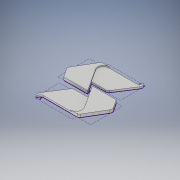
# Autodesk Inventor part: Segeco
Saved by Autodesk Inventor 2017 (Build 210142000, 142)
## iProperties
Created: 2019-09-05
Part Number: Segeco
Material: Generic
Document SubType Name: Modeling
Designer: Eduardo
Density: 1 g/cm^3
Appearance: Default
Author: Eduardo
Autodesk Inventor part; units mm, degrees
ref_plane "YZ Plane" through (0, 0, 0) normal (1, 0, 0) x (0, 1, 0)
ref_plane "XZ Plane" through (0, 0, 0) normal (0, 1, 0) x (-1, 0, 0)
ref_plane "XY Plane" through (0, 0, 0) normal (0, 0, 1) x (1, 0, 0)
sketch "SEGECO_Logo_A" plane through (0, 0, 0) normal (0, 0, 1) x (1, 0, 0)
  line L0 (106.4876, 54.7826) -> (93.1423, 75.2888)
  line L1 (131.2894, 54.7826) -> (106.4876, 54.7826)
  arc A0 (131.2894, 54.7826) -> (135.2032, 56.9315) centre (131.2894, 59.4212) ccw
  line L2 (101.453, 90.6131) -> (148.9397, 90.6131)
  arc A1 (101.453, 90.6131) -> (93.1423, 75.2888) centre (101.453, 80.6974) ccw
  line L3 (155.6383, 89.056) -> (135.2032, 56.9315)
  arc A2 (148.9397, 90.6131) -> (153.4753, 98.1434) centre (148.9397, 95.7441) ccw
  arc A3 (155.6383, 89.056) -> (153.4753, 98.1434) centre (150.146, 92.5498) ccw
  line L4 (91.5373, 98.1434) -> (156.6554, 98.1434) construction
  line L5 (156.6554, 98.1434) -> (156.6554, 54.7826) construction
  line L6 (156.6554, 54.7826) -> (91.5373, 54.7826) construction
  line L7 (91.5373, 54.7826) -> (91.5373, 98.1434) construction
  line L8 (148.9397, 90.6131) -> (148.9397, 98.1434) construction
  dimension "d53" = 9.9157
  dimension "d54" = 5.1311
  dimension "d55" = 6.5095
  dimension "d56" = 4.6386
  dimension "d63" = 1.2062
  dimension "d90" = 123.056
  dimension "d91" = 24.8018
  dimension "d92" = 20.5062
  dimension "d93" = 43.3608
  dimension "d95" = 65.1181
  measures "d53" radius of A1
  measures "d54" radius of A2
  measures "d55" radius of A3
  measures "d56" radius of A0
  measures "d63" distance from line of L8 A3.centre
  measures "d90" angle of L0 L1
  measures "d91" distance of L1.start L1.end
  measures "d92" distance from line of L0.end L6
  measures "d93" distance of L6.end L4.start
  measures "d95" distance of L4.start L4.end
sketch "SEGECO_Logo_B" plane through (0, 0, 0) normal (0, 0, 1) x (1, 0, 0)
  arc A0 (59.5618, 148.275) -> (51.2511, 132.9507) centre (59.5618, 138.3593) ccw
  line L0 (59.5618, 148.275) -> (48.761, 148.275)
  line L1 (45.0457, 146.1613) -> (26.0996, 114.2875)
  line L2 (26.2488, 108.0158) -> (35.65, 93.7862)
  line L3 (35.65, 93.7862) -> (76.7391, 93.7862)
  line L4 (76.7391, 93.7862) -> (51.2511, 132.9507)
  arc A1 (26.0996, 114.2875) -> (26.2488, 108.0158) centre (31.1752, 111.2706) ccw
  line L5 (25.2707, 148.275) -> (76.7391, 148.275) construction
  line L6 (76.7391, 148.275) -> (76.7391, 93.7862) construction
  line L7 (76.7391, 93.7862) -> (25.2707, 93.7862) construction
  line L8 (25.2707, 93.7862) -> (25.2707, 148.275) construction
  arc A2 (48.761, 148.275) -> (45.0457, 146.1613) centre (48.761, 143.9529) ccw
  point P0 (75.2707, 99.3568)
  dimension "d68" = 9.9157
  dimension "d70" = 5.9045
  dimension "d76" = 5.5706
  dimension "d77" = 1.4684
  dimension "d82" = 123.452
  dimension "d83" = 123.056
  dimension "d84" = 14.2295
  dimension "d86" = 54.4888
  dimension "d87" = 51.4684
  dimension "d89" = 23.4904
  dimension "d100" = 4.3221
  measures "d68" radius of A0
  measures "d70" radius of A1
  measures "d76" vertical distance of L3.end point (75.271, 99.357)
  measures "d77" distance from line of L6 point (75.271, 99.357)
  measures "d82" angle of L7 L2
  measures "d83" angle of L4 L7
  measures "d84" distance from line of L2.start L7
  measures "d86" distance of L7.end L5.start
  measures "d87" distance of L5.start L5.end
  measures "d89" distance of L5.start L0.end
  measures "d100" radius of A2
sketch "Logo_base" plane through (0, 0, 0) normal (0, 0, 1) x (1, 0, 0)
  arc A0 (-15.7088, 48.9181) -> (-24.0196, 33.5938) centre (-15.7088, 39.0024) ccw
  line L0 (-15.7088, 48.9181) -> (-26.5096, 48.9181)
  line L1 (-30.2249, 46.8044) -> (-49.171, 14.9307)
  line L2 (-49.0219, 8.6589) -> (-39.6206, -5.5706)
  line L3 (-39.6206, -5.5706) -> (1.4684, -5.5706)
  line L4 (1.4684, -5.5706) -> (-24.0196, 33.5938)
  arc A1 (-49.171, 14.9307) -> (-49.0219, 8.6589) centre (-44.0955, 11.9137) ccw
  line L5 (-50, 48.9181) -> (1.4684, 48.9181) construction
  line L6 (1.4684, 48.9181) -> (1.4684, -5.5706) construction
  line L7 (1.4684, -5.5706) -> (-50, -5.5706) construction
  line L8 (-50, -5.5706) -> (-50, 48.9181) construction
  arc A2 (-26.5096, 48.9181) -> (-30.2249, 46.8044) centre (-26.5096, 44.596) ccw
  line L9 (-10.6743, 13.0877) -> (-24.0196, 33.5938)
  line L10 (14.1275, 13.0877) -> (-10.6743, 13.0877)
  arc A3 (14.1275, 13.0877) -> (18.0413, 15.2366) centre (14.1275, 17.7263) ccw
  line L11 (-15.7088, 48.9181) -> (31.7778, 48.9181)
  arc A4 (-15.7088, 48.9181) -> (-24.0196, 33.5938) centre (-15.7088, 39.0024) ccw
  line L12 (38.4765, 47.361) -> (18.0413, 15.2366)
  arc A5 (31.7778, 48.9181) -> (36.3134, 56.4485) centre (31.7778, 54.0492) ccw
  arc A6 (38.4765, 47.361) -> (36.3134, 56.4485) centre (32.9841, 50.8548) ccw
  line L13 (-25.6245, 56.4485) -> (39.4935, 56.4485) construction
  line L14 (39.4935, 56.4485) -> (39.4935, 13.0877) construction
  line L15 (39.4935, 13.0877) -> (-25.6245, 13.0877) construction
  line L16 (-25.6245, 13.0877) -> (-25.6245, 56.4485) construction
  line L17 (31.7778, 48.9181) -> (31.7778, 56.4485) construction
  arc A7 (15.7088, -48.9181) -> (24.0196, -33.5938) centre (15.7088, -39.0024) ccw
  line L18 (15.7088, -48.9181) -> (26.5096, -48.9181)
  line L19 (30.2249, -46.8044) -> (49.171, -14.9307)
  line L20 (49.0219, -8.6589) -> (39.6206, 5.5706)
  line L21 (39.6206, 5.5706) -> (-1.4684, 5.5706)
  line L22 (-1.4684, 5.5706) -> (24.0196, -33.5938)
  arc A8 (49.171, -14.9307) -> (49.0219, -8.6589) centre (44.0955, -11.9137) ccw
  line L23 (50, -48.9181) -> (-1.4684, -48.9181) construction
  line L24 (-1.4684, -48.9181) -> (-1.4684, 5.5706) construction
  line L25 (-1.4684, 5.5706) -> (50, 5.5706) construction
  line L26 (50, 5.5706) -> (50, -48.9181) construction
  arc A9 (26.5096, -48.9181) -> (30.2249, -46.8044) centre (26.5096, -44.596) ccw
  line L27 (10.6743, -13.0877) -> (24.0196, -33.5938)
  line L28 (-14.1275, -13.0877) -> (10.6743, -13.0877)
  arc A10 (-14.1275, -13.0877) -> (-18.0413, -15.2366) centre (-14.1275, -17.7263) ccw
  line L29 (15.7088, -48.9181) -> (-31.7778, -48.9181)
  arc A11 (15.7088, -48.9181) -> (24.0196, -33.5938) centre (15.7088, -39.0024) ccw
  line L30 (-38.4765, -47.361) -> (-18.0413, -15.2366)
  arc A12 (-31.7778, -48.9181) -> (-36.3134, -56.4485) centre (-31.7778, -54.0492) ccw
  arc A13 (-38.4765, -47.361) -> (-36.3134, -56.4485) centre (-32.9841, -50.8548) ccw
  line L31 (25.6245, -56.4485) -> (-39.4935, -56.4485) construction
  line L32 (-39.4935, -56.4485) -> (-39.4935, -13.0877) construction
  line L33 (-39.4935, -13.0877) -> (25.6245, -13.0877) construction
  line L34 (25.6245, -13.0877) -> (25.6245, -56.4485) construction
  line L35 (-31.7778, -48.9181) -> (-31.7778, -56.4485) construction
  point P0 (0, 0)
  constraints: 2 other
extrude "Logo_A" add sketch "Logo_base" along normal blind 3 contours L11 A5 A6 L12 A3 L10 L4 A0 | L29 A12 A13 L30 A10 L28 L22 A7
extrude "Logo_B" add sketch "Logo_base" along normal blind 5 contours A0 L4 L3 L2 A1 L1 A2 L0 | A7 L22 L21 L20 A8 L19 A9 L18
equation "\"la_wdt_t\" = 65.11809"
equation "\"la_wdt_1\" = 8.20318"
equation "\"la_wdt_2\" = 24.80181"
equation "\"la_hgt_t\" = 43.36081"
equation "\"la_hgt_1\" = 20.50619"
equation "\"la_crv_1\" = 4.6386"
equation "\"la_crv_2\" = 5.13107"
equation "\"la_crv_3\" = 6.50946"
equation "\"la_d_crv_2_3\" = 1.20624"
equation "\"la_lb_crv\" = 9.9157"
equation "\"lb_crv_2\" = 4.32209"
equation "\"lb_hgt_2\" = 31.91169"
equation "\"lb_wdt_1\" = 23.49038"
equation "\"lb_wdt_2\" = 9.00605"
equation "\"lb_wdt_t\" = 51.46841"
equation "\"lb_hgt_t\" = 54.48876"
equation "\"lb_crv_1\" = 5.9045"
equation "\"lb_hgt_1\" = 14.22955"
equation "\"lb_cy\" = 5.57064"
equation "\"lb_cx\" = 1.46841"
equation "\"la_lb_ang_2\" = 56.944183deg"
equation "\"la_lb_ang_1\" = 123.055817deg"
body "Solid2"
